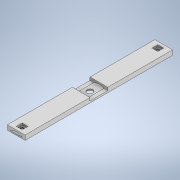
# Autodesk Inventor part: bridge1
Saved by Autodesk Inventor 2022 (Build 260153000, 153)
## iProperties
Created: 2021-10-12
Part Number: bridge1
Material: Generic
Document SubType Name: Modeling
Designer: Nikita
Density: 1 g/cm^3
Appearance: Default
Author: Nikita
Autodesk Inventor part; units mm, degrees
ref_plane "YZ Plane" through (0, 0, 0) normal (1, 0, 0) x (0, 1, 0)
ref_plane "XZ Plane" through (0, 0, 0) normal (0, 1, 0) x (-1, 0, 0)
ref_plane "XY Plane" through (0, 0, 0) normal (0, 0, 1) x (1, 0, 0)
sketch "Sketch1" plane through (0, 0, 0) normal (0, 0, 1) x (1, 0, 0)
  line L0 (0, 0) -> (30, 0)
  line L1 (30, 0) -> (30, 8)
  line L2 (30, 8) -> (0, 8)
  line L3 (0, 8) -> (0, 0)
  line L4 (14.9976, 2) -> (24.9976, 2)
  line L5 (14.9976, 2) -> (4.9976, 2)
  arc A0 (24.9976, 2) -> (4.9976, 2) centre (14.9976, -10.49) ccw
  dimension "d2" = 30
  dimension "d3" = 8
  dimension "d6" = 10
  dimension "d7" = 10
  dimension "d8" = 2
  dimension "d9" = 16
  constraints: 12 end point, 3 parallel, 2 horizontal, 2 point on circle, 1 centre point, 1 perpendicular
  measures "d2" distance of L2.end L1.end
  measures "d3" distance of L1.end L0.end
  measures "d6" distance of L4.start L4.end
  measures "d7" distance of L4.start L5.end
  measures "d8" distance from line of L0 L4.start
  measures "d9" radius of A0
extrude "Extrusion1" add sketch "Sketch1" along normal blind 250
sketch "Sketch2" plane through (0, 8, 0) normal (0, 1, 0) x (1, 0, 0)
  line L0 (30, 0) -> (0, 0) projected
  line L1 (30, 0) -> (30, -250) projected
  circle A0 centre (15, -125) radius 5
  line L2 (30, -250) -> (0, -250) projected
  line L3 (10, -15) -> (10, -5)
  line L4 (10, -5) -> (20, -5)
  line L5 (20, -5) -> (20, -15)
  line L6 (20, -15) -> (10, -15)
  line L7 (10, -15) -> (20, -5) construction
  line L8 (10, -5) -> (20, -15) construction
  line L9 (0, 0) -> (0, -250) projected
  line L10 (10, -235) -> (10, -245)
  line L11 (10, -245) -> (20, -245)
  line L12 (20, -245) -> (20, -235)
  line L13 (20, -235) -> (10, -235)
  line L14 (10, -235) -> (20, -245) construction
  line L15 (10, -245) -> (20, -235) construction
  point P0 (15, 0)
  point P1 (30, -125)
  point P2 (15, -5)
  point P3 (15, -10)
  point P4 (15, -240)
  point P5 (15, -245)
  dimension "d13" = 10
  dimension "d14" = 120
  dimension "d16" = 0
  dimension "d17" = 125
  dimension "d19" = 5
  dimension "d20" = 10
  dimension "d21" = 10
  dimension "d22" = 5
  dimension "d23" = 10
  dimension "d24" = 5
  dimension "d25" = 5
  dimension "d26" = 10
  constraints: 24 end point, 6 midpoint, 4 parallel, 2 perpendicular, 2 vertical, 1 centre point, 1 coincident
  measures "d13" diameter of A0
  measures "d14" distance of A0.centre point (15, -5)
  measures "d16" vertical distance of point (15, -125) point (30, -125)
  measures "d17" distance of point (15, 0) A0.centre
  measures "d19" distance of point (15, -5) point (15, -10)
  measures "d20" distance of L3.end L4.end
  measures "d21" distance of L3.start L3.end
  measures "d22" distance of point (15, 0) point (15, -5)
  measures "d23" distance between parallel lines of L1 L5
  measures "d24" distance from line of L2 point (15, -245)
  measures "d25" distance of point (15, -245) point (15, -240)
  measures "d26" distance of L11.end L10.end
extrude "Extrusion2" cut sketch "Sketch2" against normal up to surface (8 mm away) from surface at 0 contours A0 | L3 L4 L5 L6 | L13 L12 L11 L10
sketch "Sketch3" plane through (0, 8, 0) normal (0, 1, 0) x (1, 0, 0)
  line L0 (30, 0) -> (30, -250) projected
  line L1 (30, 0) -> (0, 0) projected
  line L2 (0, -140) -> (30, -140)
  line L3 (30, -140) -> (30, -110)
  line L4 (30, -110) -> (0, -110)
  line L5 (0, -110) -> (0, -140)
  line L6 (0, -140) -> (30, -110) construction
  line L7 (30, -140) -> (0, -110) construction
  line L8 (4.9976, 0) -> (4.9976, -250) projected
  point P0 (30, -125)
  point P1 (15, 0)
  point P2 (15, -125)
  dimension "d29" = 15
  dimension "d30" = 125
  dimension "d31" = 30
  dimension "d32" = 30
  constraints: 12 end point, 4 midpoint, 2 parallel, 2 perpendicular
  measures "d29" distance of point (15, -125) point (30, -125)
  measures "d30" distance of point (15, 0) point (15, -125)
  measures "d31" distance of L3.end L2.end
  measures "d32" distance of L3.end L4.end
extrude "Extrusion3" cut sketch "Sketch3" against normal blind 5 contours L0 L2 L8 L4 | L8 L2 L5 L4
body "Solid1"
